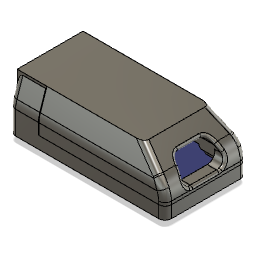
bms_can_case (Autodesk Fusion 360 design; units mm, degrees)
Autodesk Fusion 360 part; units mm, degrees
sketch "Sketch1" plane through (0, 0, 0) normal (0, 1, 0) x (1, 0, 0) in component "arduino nano"
  line L0 (0, 0) -> (44, 0)
  line L1 (44, 0) -> (44, -18)
  line L2 (44, -18) -> (0, -18)
  line L3 (0, -18) -> (0, 0)
  line L4 (0, -9) -> (-5, -9) construction
  line L5 (0, -5) -> (-5, -5)
  line L6 (0, -13) -> (-5, -13)
  line L7 (-2, -4) -> (-2, -14)
  line L8 (0, -5) -> (10, -5)
  line L9 (10, -5) -> (10, -13)
  line L10 (10, -13) -> (0, -13)
  dimension "d1571" = 44
  dimension "d1572" = 18
  dimension "d1573" = 4
  dimension "d1574" = -4
  constraint horizontal L0
  constraint vertical L1
  constraint horizontal L2
  constraint vertical L3
  constraint coincident L0.start L3.end
  constraint midpoint L3 L4.start
  constraint perpendicular L3 L4
  constraint perpendicular L6 L7
  constraint perpendicular L3 L8
  constraint perpendicular L5 L9
  measures "d1571" distance of L0.start L0.end
  measures "d1572" distance of L0.start L2.end
extrude "Extrude1" add sketch "Sketch1" along normal blind 5.7 contours L3 L8 L9 L10 | L3 L5 L6 L7 makes body 1 in component "arduino nano"
extrude "Extrude2" add sketch "Sketch1" along normal blind 1.5 contours L0 L1 L2 L3 L8 L9 L10 bodies 1 in component "arduino nano"
ref_plane "WorkPlane1" through (4, 6.2, 9) normal (0, 1, 0) x (0, 0, 1) in component "case bottom (1)"
sketch "Sketch1 (2)" plane through (4, 6.2, 9) normal (0, 1, 0) x (1, 0, 0) in component "case bottom (1)"
  line L0 (-4, 4) -> (6, 4)
  line L1 (6, 4) -> (6, -4)
  line L2 (6, -4) -> (-4, -4)
  line L3 (-4, -4) -> (-4, -9)
  line L4 (-4, -9) -> (40, -9)
  line L5 (40, -9) -> (40, 9)
  line L6 (40, 9) -> (-4, 9)
  line L7 (-4, 9) -> (-4, 4)
  line L8 (-4, 4) -> (-4, -4)
  line L9 (-8, -4) -> (-8, -13)
  line L10 (-8, -13) -> (44, -13)
  line L11 (44, -13) -> (44, 13)
  line L12 (44, 13) -> (-8, 13)
  line L13 (-8, 13) -> (-8, 4)
  line L14 (-8, 4) -> (-8, -4)
  line L15 (-4.25, -4) -> (-4.25, -9.25)
  line L16 (-4.25, -9.25) -> (40.25, -9.25)
  line L17 (40.25, -9.25) -> (40.25, 9.25)
  line L18 (40.25, 9.25) -> (-4.25, 9.25)
  line L19 (-4.25, 9.25) -> (-4.25, 4)
  line L20 (-6, 8) -> (-8, 8)
  line L21 (-6, 8) -> (-6, -8)
  line L22 (-6, -8) -> (-8, -8)
  line L23 (6, -4.5) -> (-4, -4.5) construction
  line L24 (-4, 4.5) -> (6, 4.5) construction
  line L25 (-4, 4.5) -> (-6, 4.5)
  line L26 (-4, -4.5) -> (-6, -4.5)
  dimension "d1580" = 4
  dimension "d1581" = 0.25
  dimension "d1584" = -0.5
  dimension "d1585" = -0.5
  constraint coincident L0.start L7.end
  constraint coincident L2.end L3.start
  constraint coincident L13 L20.end
  constraint perpendicular L13 L20
  constraint perpendicular L20 L21
  constraint coincident L9 L22.end
  constraint perpendicular L9 L22
  constraint coincident L21 L25.end
  constraint perpendicular L21 L25
  constraint coincident L21 L26.end
  constraint perpendicular L21 L26
extrude "Extrude1'" add sketch "Sketch1 (2)" along normal blind 0.8 separate body contours L0 L1 L2 L3 L4 L5 L6 L7 | L3 L7 L8 L21 L25 L26 | L0 L1 L2 L8 | L3 L4 L5 L6 L7 L15 L16 L17 L18 L19 L25 L26 | L9 L10 L11 L12 L13 L15 L16 L17 L18 L19 L20 L21 L22 L25 L26 makes body 2 in component "case bottom (1)"
extrude "Extrude2'" add sketch "Sketch1 (2)" against normal blind 6.5 contours L9 L10 L11 L12 L13 L15 L16 L17 L18 L19 L20 L21 L22 L25 L26 bodies 2 in component "case bottom (1)"
sketch "Sketch2" plane through (0, 6.2, 0) normal (0, -1, 0) x (1, 0, 0) in component "case bottom (1)"
  line L0 (-2, 4.5) -> (-0.25, 4.5)
  line L1 (-0.25, 4.5) -> (-0.25, -0.25)
  line L2 (-0.25, -0.25) -> (44.25, -0.25)
  line L3 (44.25, -0.25) -> (44.25, 18.25)
  line L4 (44.25, 18.25) -> (-0.25, 18.25)
  line L5 (-0.25, 18.25) -> (-0.25, 13.5)
  line L6 (-0.25, 13.5) -> (-2, 13.5)
  line L7 (-2, 13.5) -> (-2, 4.5)
  line L8 (2.25, 4.5) -> (2.25, 2.25) construction
  line L9 (2.25, 2.25) -> (41.75, 2.25) construction
  line L10 (41.75, 2.25) -> (41.75, 15.75) construction
  line L11 (41.75, 15.75) -> (2.25, 15.75) construction
  line L12 (2.25, 15.75) -> (2.25, 13.5) construction
  line L13 (2.25, 2.25) -> (2.25, -0.25)
  line L14 (2.25, 2.25) -> (-0.25, 2.25)
  line L15 (-0.25, 2.25) -> (-0.25, -0.25)
  line L16 (-0.25, -0.25) -> (2.25, -0.25)
  line L17 (2.25, 15.75) -> (-0.25, 15.75)
  line L18 (-0.25, 15.75) -> (-0.25, 18.25)
  line L19 (-0.25, 18.25) -> (2.25, 18.25)
  line L20 (2.25, 18.25) -> (2.25, 15.75)
  line L21 (41.75, 15.75) -> (44.25, 15.75)
  line L22 (44.25, 15.75) -> (44.25, 18.25)
  line L23 (44.25, 18.25) -> (41.75, 18.25)
  line L24 (41.75, 18.25) -> (41.75, 15.75)
  line L25 (41.75, 2.25) -> (44.25, 2.25)
  line L26 (44.25, 2.25) -> (44.25, -0.25)
  line L27 (44.25, -0.25) -> (41.75, -0.25)
  line L28 (41.75, -0.25) -> (41.75, 2.25)
  dimension "d1588" = -2.5
  constraint coincident L2 L13.end
  constraint perpendicular L2 L13
  constraint coincident L1 L14.end
  constraint perpendicular L1 L14
  constraint coincident L1.end L2.start
  constraint horizontal L17
  constraint vertical L18
  constraint horizontal L19
  constraint vertical L20
  constraint coincident L4.end L5.start
  constraint horizontal L21
  constraint vertical L22
  constraint horizontal L23
  constraint vertical L24
  constraint coincident L3.end L4.start
  constraint horizontal L25
  constraint vertical L26
  constraint horizontal L27
  constraint vertical L28
  constraint coincident L2.end L3.start
extrude "Extrude3" add sketch "Sketch2" along normal blind 4.5 contours L1 L2 L13 L14 L15 L16 | L4 L5 L17 L18 L19 L20 | L2 L3 L25 L26 L27 L28 | L3 L4 L21 L22 L23 L24 bodies 2 in component "case bottom (1)"
sketch "Sketch3" plane through (0, -0.3, 0) normal (0, -1, 0) x (1, 0, 0) in component "case bottom (1)"
  line L0 (-2, 17) -> (-2, 13.5)
  line L1 (-2, 13.5) -> (-0.25, 13.5)
  line L2 (-0.25, 13.5) -> (-0.25, 18.25)
  line L3 (-0.25, 18.25) -> (44.25, 18.25)
  line L4 (44.25, 18.25) -> (44.25, -0.25)
  line L5 (44.25, -0.25) -> (-0.25, -0.25)
  line L6 (-0.25, -0.25) -> (-0.25, 4.5)
  line L7 (-0.25, 4.5) -> (-2, 4.5)
  line L8 (-2, 4.5) -> (-2, 1)
  line L9 (-2, 1) -> (-4, 1)
  line L10 (-4, 1) -> (-4, -4)
  line L11 (-4, -4) -> (48, -4)
  line L12 (48, -4) -> (48, 22)
  line L13 (48, 22) -> (-4, 22)
  line L14 (-4, 22) -> (-4, 17)
  line L15 (-4, 17) -> (-2, 17)
  line L16 (9.75, 13.5) -> (9.75, 18.25) construction
  line L17 (9.75, 18.25) -> (9.75, 22)
  line L18 (9.75, 18.25) -> (9.75, -4)
  dimension "d1591" = 10
  constraint coincident L13 L17.end
  constraint perpendicular L13 L17
  constraint coincident L11 L18.end
  constraint perpendicular L11 L18
extrude "Extrude4" add sketch "Sketch3" along normal blind 4 contours L3 L4 L5 L11 L12 L13 L17 L18 bodies 2 in component "case bottom (1)"
ref_plane "WorkPlane1" through (22, -7, 9) normal (0, 1, 0) x (1, 0, 0) in component "mcp2515"
sketch "Sketch1 (3)" plane through (22, -7, 9) normal (0, 1, 0) x (1, 0, 0) in component "mcp2515"
  line L0 (-22, -9) -> (-22, 9) construction
  line L1 (-7.5, -9) -> (-7.5, 9) construction
  line L2 (-9, 0) -> (-6, 0) construction
  line L3 (-9, -13.85) -> (-6, -13.85) construction
  line L4 (-9, 13.85) -> (-6, 13.85) construction
  line L5 (-7.5, -9) -> (-7.5, -13.85) construction
  line L6 (-7.5, 9) -> (-7.5, 13.85) construction
  line L7 (-7.5, -13.85) -> (-7.5, 13.85)
  line L8 (32.5, -13.85) -> (32.5, 13.85)
  line L9 (-7.5, -13.85) -> (32.5, -13.85)
  line L10 (-7.5, 13.85) -> (32.5, 13.85)
  line L11 (-0.5, -13.85) -> (-0.5, 13.85) construction
  line L12 (5.35, -13.85) -> (5.35, 13.85) construction
  line L13 (-0.5, 0) -> (5.35, 0) construction
  line L14 (-0.5, -3.75) -> (5.35, -3.75)
  line L15 (-0.5, 3.75) -> (5.35, 3.75)
  line L16 (5.35, -3.75) -> (5.35, 3.75)
  line L17 (-0.5, -3.75) -> (-0.5, 3.75)
  line L18 (-5.5, -11.85) -> (32.5, -11.85) construction
  line L19 (-5.5, -11.85) -> (-5.5, 11.85) construction
  line L20 (-5.5, 11.85) -> (32.5, 11.85) construction
  line L21 (30.5, -13.85) -> (30.5, 13.85) construction
  circle A0 centre (30.5, -11.85) radius 1.65
  circle A1 centre (30.5, 11.85) radius 1.65
  circle A2 centre (-5.5, -11.85) radius 1.65
  circle A3 centre (-5.5, 11.85) radius 1.65
  dimension "d1595" = 14.5
  dimension "d1596" = 13.85
  dimension "d1597" = -13.85
  dimension "d1598" = 40
  dimension "d1599" = 7
  dimension "d1600" = 12.85
  dimension "d1601" = 3.75
  dimension "d1602" = -3.75
  dimension "d1603" = 2
  dimension "d1604" = 38
  dimension "d1605" = 3.3
  dimension "d1606" = 3.3
  dimension "d1607" = 3.3
  dimension "d1608" = 3.3
  constraint perpendicular L1 L2
  constraint midpoint L3 L5.end
  constraint midpoint L4 L6.end
  constraint perpendicular L3 L7
  constraint parallel L4 L10
  constraint midpoint L11 L13.start
  constraint midpoint L12 L13.end
  constraint perpendicular L12 L13
  constraint perpendicular L15 L16
  constraint perpendicular L15 L17
  constraint coincident L18 A0.centre
  constraint coincident L21 A0.centre
  constraint coincident L21 A1.centre
  constraint coincident L20 A1.centre
  constraint coincident L18.start L19.start
  constraint coincident L19.end L20.start
  measures "d1605" diameter of A0
  measures "d1606" diameter of A1
  measures "d1607" diameter of A2
  measures "d1608" diameter of A3
extrude "Extrude1''" add sketch "Sketch1 (3)" against normal blind 1.2 separate body contours L7 L8 L9 L10 | L14 L15 L16 L17 makes body 3 in component "mcp2515"
extrude "Extrude2''" add sketch "Sketch1 (3)" against normal blind 8.5 contours L14 L15 L16 L17 bodies 3 in component "mcp2515"
sketch "Sketch4" plane through (0, -4.3, 0) normal (0, -1, 0) x (1, 0, 0) in component "case bottom (1)"
  line L0 (9.75, 18.25) -> (44.25, 18.25)
  line L1 (44.25, 18.25) -> (44.25, -0.25)
  line L2 (44.25, -0.25) -> (9.75, -0.25)
  line L3 (9.75, -0.25) -> (9.75, -4)
  line L4 (9.75, -4) -> (48, -4)
  line L5 (48, -4) -> (48, 22)
  line L6 (48, 22) -> (9.75, 22)
  line L7 (9.75, 22) -> (9.75, 18.25)
  line L8 (14.5, -4.85) -> (54.5, -4.85) construction
  line L9 (14.5, 22.85) -> (14.5, -4.85) construction
  line L10 (54.5, 22.85) -> (54.5, -4.85) construction
  line L11 (14.5, 22.85) -> (54.5, 22.85) construction
  line L12 (54.75, 23.1) -> (54.75, -5.1)
  line L13 (14.25, -5.1) -> (54.75, -5.1)
  line L14 (14.25, 23.1) -> (14.25, -5.1)
  line L15 (14.25, 23.1) -> (54.75, 23.1)
  line L16 (14.5, -7.1) -> (59.5, -7.1)
  line L17 (14.5, 25.1) -> (59.5, 25.1)
  line L18 (54.5, -7.1) -> (54.5, 25.1) construction
  line L19 (59.5, -7.1) -> (59.5, 25.1)
  line L20 (9.75, 22) -> (9.75, 25.1)
  line L21 (9.75, 25.1) -> (14.5, 25.1)
  line L22 (14.25, 18.25) -> (9.75, 18.25)
  line L23 (9.75, 18.25) -> (9.75, 22)
  line L24 (14.5, -7.1) -> (9.75, -7.1)
  line L25 (9.75, -7.1) -> (9.75, -0.25)
  dimension "d1613" = 0.25
  dimension "d1616" = 5
  constraint perpendicular L17 L18
  constraint parallel L11 L17
  constraint coincident L18.end L17
  constraint parallel L8 L16
  constraint coincident L18.start L16
  constraint coincident L6.end L7.start
  constraint perpendicular L6 L20
  constraint perpendicular L7 L21
  constraint coincident L14 L22.start
  constraint coincident L0 L22.start
  constraint coincident L0.start L7.end
  constraint perpendicular L20 L24
  constraint coincident L2.end L3.start
  constraint perpendicular L2 L25
extrude "Extrude5" add sketch "Sketch4" along normal mid plane 4 contours L0 L6 L7 L14 L22 L23 | L4 L6 L12 L13 L14 L15 L16 L17 L19 L20 L21 L24 L25 | L4 L5 L6 L12 L13 L14 L15 | L2 L3 L4 L14 L25 bodies 2 in component "case bottom (1)"
extrude "Extrude6" add sketch "Sketch4" along normal blind 4 contours L0 L6 L7 L14 L22 L23 | L4 L6 L12 L13 L14 L15 L16 L17 L19 L20 L21 L24 L25 | L2 L3 L4 L14 L25 bodies 2 in component "case bottom (1)"
sketch "Sketch6" plane through (0, -7, 0) normal (0, 1, 0) x (-1, 0, 0) in component "case bottom (1)"
  circle A0 centre (-52.5, -2.85) radius 1.65
  circle A1 centre (-52.5, 20.85) radius 1.65
  circle A2 centre (-16.5, -2.85) radius 1.65
  circle A3 centre (-16.5, 20.85) radius 1.65
  line L0 (-14.5, 22.85) -> (-54.5, 22.85)
  line L1 (-54.5, 22.85) -> (-54.5, -4.85)
  line L2 (-54.5, -4.85) -> (-14.5, -4.85)
  line L3 (-14.5, -4.85) -> (-14.5, 22.85)
  circle A4 centre (-16.5, 20.85) radius 1.65 construction
  circle A5 centre (-52.5, 20.85) radius 1.65 construction
  circle A6 centre (-52.5, -2.85) radius 1.65 construction
  circle A7 centre (-16.5, -2.85) radius 1.65 construction
  line L4 (-14.25, 18.25) -> (-14.25, 23.1)
  line L5 (-14.25, 23.1) -> (-54.75, 23.1)
  line L6 (-54.75, 23.1) -> (-54.75, -5.1)
  line L7 (-54.75, -5.1) -> (-14.25, -5.1)
  line L8 (-14.25, -5.1) -> (-14.25, -0.25)
  line L9 (-14.25, 18.25) -> (-19, 18.25)
  line L10 (-19, 18.25) -> (-19, 23.1)
  line L11 (-14.25, -0.25) -> (-19, -0.25)
  line L12 (-19, -0.25) -> (-19, -5.1)
  line L13 (-49.9, 23.1) -> (-49.9, -5.1)
  line L14 (-19, 18.25) -> (-54.75, 18.25)
  line L15 (-19, -0.25) -> (-54.75, -0.25)
  circle A8 centre (-16.5, 20.85) radius 1
  circle A9 centre (-52.5, 20.85) radius 1
  circle A10 centre (-52.5, -2.85) radius 1
  circle A11 centre (-16.5, -2.85) radius 1
  dimension "d1621" = -4.85
  dimension "d1624" = 2
  dimension "d1625" = 2
  dimension "d1626" = 2
  dimension "d1627" = 2
  constraint coincident L4.start L9.start
  constraint perpendicular L3 L9
  constraint coincident L5 L10.end
  constraint perpendicular L5 L10
  constraint coincident L8.end L11.start
  constraint perpendicular L3 L11
  constraint perpendicular L2 L12
  constraint coincident L7 L12.end
  constraint coincident L6 L14.end
  constraint perpendicular L6 L14
  constraint coincident L6 L15.end
  constraint perpendicular L6 L15
  constraint concentric A4 A8
  constraint concentric A5 A9
  constraint concentric A6 A10
  constraint concentric A7 A11
  measures "d1624" diameter of A8
  measures "d1625" diameter of A9
  measures "d1626" diameter of A10
  measures "d1627" diameter of A11
extrude "Extrude7" add sketch "Sketch6" along normal blind 3.039 contours A0 | A1 | A2 | A3 | L0 L3 L9 L10 | L0 L3 L4 L5 L9 L10 | L0 L1 L13 L14 | L0 L1 L5 L6 L13 L14 | L2 L3 L7 L8 L11 L12 | L2 L3 L11 L12 | L1 L2 L13 L15 | L1 L2 L6 L7 L13 L15 | A8 | A9 | A10 | A11 bodies 2 in component "case bottom (1)"
extrude "Extrude8" cut sketch "Sketch6" along normal blind 3 contours A8 | A9 | A10 | A11 bodies 2 in component "case bottom (1)"
sketch "Sketch7" plane through (59.5, 0, 0) normal (1, 0, 0) x (0, 0, -1) in component "case bottom (1)"
  line L0 (7.1, -8.3) -> (7.1, -2.3)
  line L1 (7.1, -2.3) -> (-25.1, -2.3)
  line L2 (-25.1, -2.3) -> (-25.1, -8.3)
  line L3 (-25.1, -8.3) -> (7.1, -8.3)
  line L4 (-25.1, -2.3) -> (7.1, -2.3)
  line L5 (-22, -2.3) -> (-22, 7)
  line L6 (4, -2.3) -> (4, 7)
  line L7 (4, 7) -> (7.1, -2.3)
  line L8 (-25.1, -2.3) -> (-22, 7)
  constraint coincident L6.end L7.start
  constraint coincident L0.end L1.start
  constraint coincident L1.end L2.start
  constraint coincident L5.end L8.end
extrude "Extrude9" add sketch "Sketch7" against normal blind 49.75 contours L1 L4 L6 L7 | L1 L4 L5 L8 bodies 2 in component "case bottom (1)"
ref_plane "WorkPlane1" through (59.5, -2.3, -4) normal (0.628809, 0.77756, 0) x (-0.77756, 0.628809, 0) in component "case bottom (1)"
split "Split1" by plane through (59.5, -2.3, -4) normal (0.628809, 0.77756, 0) bodies 2 makes body 4 at (55.6667, 3.9, -5.0333) makes body 5 at (55.6667, 3.9, 23.0333) in component "case bottom (1)"
delete_body "RemoveBody1" bodies 4 in component "case bottom (1)"
delete_body "RemoveBody2" bodies 5 in component "case bottom (1)"
extrude "Extrude10" add 1 faces at (51.8333, 0.8, -4) along direction (0, 0, 1) blind 26 on bodies 2 bodies 2 in component "case bottom (1)"
sketch "Sketch8" plane through (44.25, 0, 0) normal (-1, 0, 0) x (0, 0, 1) in component "case bottom (1)"
  line L0 (2.25, 1.7) -> (-0.25, 1.7)
  line L1 (-0.25, 1.7) -> (-0.25, -4.3)
  line L2 (-0.25, -4.3) -> (18.25, -4.3)
  line L3 (18.25, -4.3) -> (18.25, 1.7)
  line L4 (18.25, 1.7) -> (15.75, 1.7)
  line L5 (15.75, 1.7) -> (15.75, 6.2)
  line L6 (15.75, 6.2) -> (2.25, 6.2)
  line L7 (2.25, 6.2) -> (2.25, 1.7)
  line L8 (15.75, 1.7) -> (2.25, 1.7)
  line L9 (-0.25, -6.3) -> (2.25, 1.7)
  line L10 (-0.25, -6.3) -> (18.25, -6.3)
  line L11 (18.25, -6.3) -> (15.75, 1.7)
  point P0 (18.25, -6.3)
  point P1 (-0.25, -6.3)
  point P2 (15.75, 1.7)
  point P3 (2.25, 1.7)
  constraint coincident P2 L4.end
  constraint coincident P3 L0.start
  constraint coincident P1 L9.start
  constraint coincident P0 L10.end
extrude "Extrude11" cut sketch "Sketch8" against normal blind 18.998 contours L2 L8 L9 L11 | L2 L9 L10 L11 bodies 2 in component "case bottom (1)"
sketch "Sketch1 (4)" plane through (0, -8.3, 0) normal (0, -1, 0) x (1, 0, 0) in component "case top (1)"
  line L0 (14.5, -7.1) -> (59.5, -7.1)
  line L1 (59.5, -7.1) -> (59.5, 25.1)
  line L2 (59.5, 25.1) -> (9.75, 25.1)
  line L3 (9.75, 25.1) -> (9.75, 22)
  line L4 (9.75, 22) -> (9.75, 18.25)
  line L5 (9.75, 18.25) -> (14.25, 18.25)
  line L6 (14.25, 18.25) -> (14.25, 23.1)
  line L7 (14.25, 23.1) -> (54.75, 23.1)
  line L8 (54.75, 23.1) -> (54.75, -5.1)
  line L9 (54.75, -5.1) -> (14.25, -5.1)
  line L10 (14.25, -5.1) -> (14.25, -0.25)
  line L11 (14.25, -0.25) -> (9.75, -0.25)
  line L12 (9.75, -0.25) -> (9.75, -7.1)
  line L13 (9.75, -7.1) -> (14.5, -7.1)
extrude "Extrude1'''" add sketch "Sketch1 (4)" along normal blind 4 separate body makes body 6 in component "case top (1)"
sketch "Sketch2 (2)" plane through (0, -12.3, 0) normal (0, -1, 0) x (1, 0, 0) in component "case top (1)"
  line L0 (9.75, -7.1) -> (14.5, -7.1)
  line L1 (14.5, -7.1) -> (59.5, -7.1)
  line L2 (59.5, -7.1) -> (59.5, 25.1)
  line L3 (59.5, 25.1) -> (9.75, 25.1)
  line L4 (9.75, 25.1) -> (9.75, 22)
  line L5 (9.75, 22) -> (9.75, 18.25)
  line L6 (9.75, 18.25) -> (14.25, 18.25)
  line L7 (14.25, 18.25) -> (14.25, 23.1)
  line L8 (14.25, 23.1) -> (54.75, 23.1)
  line L9 (54.75, 23.1) -> (54.75, -5.1)
  line L10 (54.75, -5.1) -> (14.25, -5.1)
  line L11 (14.25, -5.1) -> (14.25, -0.25)
  line L12 (14.25, -0.25) -> (9.75, -0.25)
  line L13 (9.75, -0.25) -> (9.75, -7.1)
  line L14 (27.35, 5.25) -> (27.35, 12.75)
  line L15 (27.35, 12.75) -> (21.5, 12.75)
  line L16 (21.5, 12.75) -> (21.5, 5.25)
  line L17 (21.5, 5.25) -> (27.35, 5.25)
  line L18 (28.35, 13.75) -> (20.5, 13.75)
  line L19 (20.5, 13.75) -> (20.5, 4.25)
  line L20 (20.5, 4.25) -> (28.35, 4.25)
  line L21 (28.35, 4.25) -> (28.35, 13.75)
  line L22 (9.75, 18.25) -> (9.75, -0.25)
  dimension "d1640" = 1
  constraint coincident L5.end L6.start
  constraint coincident L12.end L13.start
extrude "Extrude2'''" add sketch "Sketch2 (2)" along normal blind 0.8 contours L0 L1 L2 L3 L4 L5 L6 L7 L8 L9 L10 L11 L12 L13 | L6 L7 L8 L9 L10 L11 L12 L22 bodies 6 in component "case top (1)"
sketch "Sketch3 (2)" plane through (0, -12.3, 0) normal (0, 1, 0) x (-1, 0, 0) in component "case top (1)"
  line L0 (-14.25, -0.25) -> (-9.75, -0.25)
  line L1 (-9.75, -0.25) -> (-9.75, 18.25)
  line L2 (-9.75, 18.25) -> (-14.25, 18.25)
  line L3 (-14.25, 18.25) -> (-14.25, 23.1)
  line L4 (-14.25, 23.1) -> (-54.75, 23.1)
  line L5 (-54.75, 23.1) -> (-54.75, -5.1)
  line L6 (-54.75, -5.1) -> (-14.25, -5.1)
  line L7 (-14.25, -5.1) -> (-14.25, -0.25)
  line L8 (-28.35, 4.25) -> (-28.35, 13.75)
  line L9 (-28.35, 13.75) -> (-20.5, 13.75)
  line L10 (-20.5, 13.75) -> (-20.5, 4.25)
  line L11 (-20.5, 4.25) -> (-28.35, 4.25)
  line L12 (-14.25, -0.25) -> (-14.25, 18.25)
  constraint coincident L0.start L7.end
  constraint coincident L2.end L3.start
extrude "Extrude3'" add sketch "Sketch3 (2)" along normal blind 7 contours L0 L1 L2 L12 bodies 6 in component "case top (1)"
extrude "Extrude4'" cut 1 faces at (12.75, -6.3, 18.25) along direction (0, 0, -1) blind 0.25 on bodies 6 bodies 6 in component "case top (1)"
extrude "Extrude5'" cut 1 faces at (11.25, -6.3, -0.25) along direction (0, 0, 1) blind 0.25 on bodies 6 bodies 6 in component "case top (1)"
chamfer "Chamfer1" distance 2 distance2 3 1 edges at (14.25, -5.3, 9) measured on face at (11.25, -5.3, 12) on bodies 6 in component "case top (1)"
fillet "Fillet1" radius 3 4 edges at (34.5, -12.3, -5.1) (54.75, -12.3, 9) (34.5, -12.3, 23.1) (14.25, -12.3, 9) on bodies 6 in component "case top (1)"
sketch "Sketch4 (2)" plane through (0, -13.1, 0) normal (0, -1, 0) x (1, 0, 0) in component "case top (1)"
  line L0 (28.35, 13.75) -> (28.35, 4.25)
  line L1 (28.35, 4.25) -> (20.5, 4.25)
  line L2 (20.5, 4.25) -> (20.5, 13.75)
  line L3 (20.5, 13.75) -> (28.35, 13.75)
  line L4 (9.75, 22) -> (9.75, -7.1)
  line L5 (9.75, -7.1) -> (14.5, -7.1)
  line L6 (14.5, -7.1) -> (59.5, -7.1)
  line L7 (59.5, -7.1) -> (59.5, 25.1)
  line L8 (59.5, 25.1) -> (9.75, 25.1)
  line L9 (9.75, 25.1) -> (9.75, 22)
  line L10 (12.75, 22) -> (12.75, -4.1) construction
  line L11 (12.75, -4.1) -> (14.5, -4.1) construction
  line L12 (14.5, -4.1) -> (56.5, -4.1) construction
  line L13 (56.5, -4.1) -> (56.5, 22.1) construction
  line L14 (56.5, 22.1) -> (12.75, 22.1) construction
  line L15 (12.75, 22.1) -> (12.75, 22) construction
  circle A0 centre (12.75, 22.1) radius 2
  circle A1 centre (12.75, -4.1) radius 2
  circle A2 centre (56.5, -4.1) radius 2
  circle A3 centre (56.5, 22.1) radius 2
  circle A4 centre (12.75, 22.1) radius 1.25
  circle A5 centre (12.75, -4.1) radius 1.25
  circle A6 centre (56.5, 22.1) radius 1.25
  circle A7 centre (56.5, -4.1) radius 1.25
  dimension "d1653" = -3
  dimension "d1654" = 4
  dimension "d1655" = 4
  dimension "d1656" = 4
  dimension "d1657" = 4
  dimension "d1658" = 2.5
  dimension "d1659" = 2.5
  dimension "d1660" = 2.5
  dimension "d1661" = 2.5
  constraint coincident L14.end L15.start
  constraint coincident L10.end L11.start
  constraint coincident L12.end L13.start
  constraint coincident L13.end L14.start
  constraint concentric A0 A4
  constraint concentric A2 A7
  measures "d1654" diameter of A0
  measures "d1655" diameter of A1
  measures "d1656" diameter of A2
  measures "d1657" diameter of A3
  measures "d1658" diameter of A4
  measures "d1659" diameter of A5
  measures "d1660" diameter of A6
  measures "d1661" diameter of A7
extrude "Extrude6'" cut sketch "Sketch4 (2)" against normal blind 2 contours A0 | A1 | A2 | A3 bodies 6 in component "case top (1)"
extrude "Extrude7'" cut 4 faces at (13.1482, -13.1, 21.8612) (56.2402, -13.1, 21.65) (56.6522, -13.1, -4.3637) (12.4822, -13.1, -3.5672) along direction (0, 1, 0) blind 7.362 on bodies 6 bodies 6 in component "case top (1)"
sketch "Sketch5" plane through (9.75, 0, 0) normal (-1, 0, 0) x (0, 0, 1) in component "case top (1)"
  line L0 (0, -8.3) -> (-7.1, -8.3)
  line L1 (-7.1, -8.3) -> (-7.1, -13.1)
  line L2 (-7.1, -13.1) -> (22, -13.1)
  line L3 (22, -13.1) -> (22, -8.3)
  line L4 (22, -8.3) -> (18, -8.3)
  line L5 (18, -8.3) -> (18, -5.3)
  line L6 (18, -5.3) -> (0, -5.3)
  line L7 (0, -5.3) -> (0, -8.3)
  line L8 (25.1, -8.3) -> (22, -8.3)
  line L9 (22, -8.3) -> (22, -13.1)
  line L10 (22, -13.1) -> (25.1, -13.1)
  line L11 (25.1, -13.1) -> (25.1, -8.3)
extrude "Extrude8'" add sketch "Sketch5" along normal blind 0.25 bodies 6 in component "case top (1)"
sketch "Sketch6 (2)" plane through (9.5, 0, 0) normal (-1, 0, 0) x (0, 0, 1) in component "case top (1)"
  line L0 (25.1, -13.1) -> (25.1, -8.3)
  line L1 (25.1, -8.3) -> (18, -8.3)
  line L2 (18, -8.3) -> (18, -5.3)
  line L3 (18, -5.3) -> (0, -5.3)
  line L4 (0, -5.3) -> (0, -8.3)
  line L5 (0, -8.3) -> (-7.1, -8.3)
  line L6 (-7.1, -8.3) -> (-7.1, -13.1)
  line L7 (-7.1, -13.1) -> (25.1, -13.1)
  line L8 (-0.25, -8.3) -> (-0.25, -0.3) construction
  line L9 (-0.25, -0.3) -> (-4, -0.3) construction
  line L10 (-4, -0.3) -> (-4, 7) construction
  line L11 (-4, 7) -> (-7.1, -2.3) construction
  line L12 (-7.1, -2.3) -> (-7.1, -8.3) construction
  line L13 (-7.1, -8.3) -> (-0.25, -8.3) construction
  line L14 (25.1, -8.3) -> (25.1, -2.3) construction
  line L15 (25.1, -2.3) -> (22, -2.3) construction
  line L16 (22, -2.3) -> (22, -8.3) construction
  line L17 (22, -8.3) -> (25.1, -8.3) construction
  line L18 (22, -8.3) -> (22, -2.3) construction
  line L19 (22, -2.3) -> (25.1, -2.3) construction
  line L20 (25.1, -2.3) -> (22, 7) construction
  line L21 (22, 7) -> (22, -0.3) construction
  line L22 (22, -0.3) -> (18.25, -0.3) construction
  line L23 (18.25, -0.3) -> (18.25, -8.3) construction
  line L24 (18.25, -8.3) -> (22, -8.3) construction
  line L25 (-0.25, -0.55) -> (-4.25, -0.55) construction
  line L26 (-4.25, -0.55) -> (-4.25, 7) construction
  line L27 (22.25, 7) -> (22.25, -0.55) construction
  line L28 (22.25, -0.55) -> (18.25, -0.55) construction
  line L29 (25.1, -13.1) -> (-7.1, -13.1)
  line L30 (-7.1, -2.3) -> (-4.25, 6.25)
  line L31 (-7.1, -2.3) -> (-7.1, -13.1)
  line L32 (-4.25, 6.25) -> (-4.25, -0.55)
  line L33 (-4.25, -0.55) -> (0, -0.55)
  line L34 (0, -0.55) -> (0, -5.3)
  line L35 (25.1, -13.1) -> (25.1, -2.3)
  line L36 (25.1, -2.3) -> (22.25, 6.25)
  line L37 (22.25, 6.25) -> (22.25, -0.55)
  line L38 (22.25, -0.55) -> (18, -0.55)
  line L39 (18, -0.55) -> (18, -5.3)
  dimension "d1692" = -0.25
  dimension "d1693" = -0.25
  constraint coincident L0.start L7.end
  constraint coincident L6.end L7.start
  constraint coincident L11.end L12.start
  constraint coincident L11 L30.end
  constraint coincident L26 L30.end
  constraint perpendicular L8 L33
  constraint coincident L3.end L4.start
  constraint perpendicular L3 L34
  constraint coincident L14.end L15.start
  constraint coincident L20 L36.end
  constraint coincident L27 L36.end
  constraint perpendicular L23 L38
  constraint coincident L2.end L3.start
extrude "Extrude9'" add sketch "Sketch6 (2)" along normal blind 11.5 bodies 6 in component "case top (1)"
sketch "Sketch9" plane through (0, -8.3, 0) normal (0, -1, 0) x (1, 0, 0) in component "case bottom (1)"
  line L0 (14.5, -7.1) -> (59.5, -7.1)
  line L1 (59.5, -7.1) -> (59.5, 25.1)
  line L2 (59.5, 25.1) -> (9.75, 25.1)
  line L3 (9.75, 25.1) -> (9.75, 22)
  line L4 (9.75, 22) -> (9.75, 18.25)
  line L5 (9.75, 18.25) -> (14.25, 18.25)
  line L6 (14.25, 18.25) -> (14.25, 23.1)
  line L7 (14.25, 23.1) -> (54.75, 23.1)
  line L8 (54.75, 23.1) -> (54.75, -5.1)
  line L9 (54.75, -5.1) -> (14.25, -5.1)
  line L10 (14.25, -5.1) -> (14.25, -0.25)
  line L11 (14.25, -0.25) -> (9.75, -0.25)
  line L12 (9.75, -0.25) -> (9.75, -7.1)
  line L13 (9.75, -7.1) -> (14.5, -7.1)
  circle A0 centre (12.75, 22.1) radius 1.25 construction
  circle A1 centre (56.5, 22.1) radius 1.25 construction
  circle A2 centre (56.5, -4.1) radius 1.25 construction
  circle A3 centre (12.75, -4.1) radius 1.25 construction
  circle A4 centre (12.75, 22.1) radius 1
  circle A5 centre (12.75, -4.1) radius 1
  circle A6 centre (56.5, 22.1) radius 1
  circle A7 centre (56.5, -4.1) radius 1
  dimension "d1672" = 2
  dimension "d1673" = 2
  dimension "d1674" = 2
  dimension "d1675" = 2
  constraint concentric A0 A4
  constraint concentric A3 A5
  constraint concentric A1 A6
  constraint concentric A2 A7
  measures "d1672" diameter of A4
  measures "d1673" diameter of A5
  measures "d1674" diameter of A6
  measures "d1675" diameter of A7
extrude "Extrude12" cut sketch "Sketch9" against normal blind 4 contours A4 | A5 | A6 | A7 bodies 2 in component "case bottom (1)"
fillet "Fillet2" radius 3 2 edges at (49.4019, 1.7, 15.75) (49.4019, 1.7, 2.25) on bodies 2 in component "case bottom (1)"
fillet "Fillet3" radius 3 2 edges at (57.125, -6.3, -0.25) (57.125, -6.3, 18.25) on bodies 2 in component "case bottom (1)"
fillet "Fillet4" radius 10 5 edges at (37, -2.3, -7.1) (12.125, -2.3, -7.1) (59.5, -2.3, -3.05) (59.5, -2.3, 21.05) (34.625, -2.3, 25.1) on bodies 2 in component "case bottom (1)"
fillet "Fillet5" radius 2.5 10 edges at (59.5, -7.6869, -7.1) (59.3718, -5.4778, -7.1) (58.2593, -2.2493, -6.959) (56.5596, 0.0087, -6.3304) (51.894, 3.8509, -5.0497) (59.5, -7.6869, 25.1) (59.3718, -5.4778, 25.1) (58.2731, -2.2747, 24.9632) (56.5596, 0.0087, 24.3304) (51.894, 3.8509, 23.0497) on bodies 2 in component "case bottom (1)"
extrude "Extrude13" cut 1 faces at (-2.6667, 2.1333, 17) along direction (0, 0, 1) blind 11.404 on bodies 2 bodies 2 in component "case bottom (1)"
extrude "Extrude14" cut 1 faces at (-2.6667, 2.1333, 1) along direction (0, 0, -1) blind 11.066 on bodies 2 bodies 2 in component "case bottom (1)"
fillet "Fillet5'" radius 10 2 edges at (3.75, -2.3, -7.1) (3.75, -2.3, 25.1) on bodies 6 in component "case top (1)"
fillet "Fillet10" radius 2.5 6 edges at (-2, 2.7448, -5.4184) (-2, -2.321, -6.9709) (-2, -8.5114, -7.1) (-2, -8.5114, 25.1) (-2, -2.321, 24.9709) (-2, 2.7448, 23.4184) on bodies 6 in component "case top (1)"
fillet "Fillet11" radius 2.5 2 edges at (59.5, -10.7, -7.1) (59.5, -10.7, 25.1) on bodies 6 in component "case top (1)"
fillet "Fillet13" radius 2.5 2 edges at (3.75, -5.3, 0) (3.75, -5.3, 18) on bodies 6 in component "case top (1)"
fillet "Fillet6" radius 1 10 edges at (59.47, -6.3, 9) (59.2859, -5.0163, 16.6289) (57.7087, -1.3626, 16.7071) (56.3733, 0.1896, 16.1484) (54.8764, 1.4391, 14.7681) (54.5538, 1.7, 9) (54.8764, 1.4391, 3.2319) (56.3733, 0.1896, 1.8516) (57.7087, -1.3626, 1.2929) (59.2859, -5.0163, 1.3711) on bodies 2 in component "case bottom (1)"
fillet "Fillet14" radius 1 5 edges at (-2, -1.675, 18) (-2, -4.5678, 17.2678) (-2, -5.3, 9) (-2, -4.5678, 0.7322) (-2, -1.675, 0) on bodies 6 in component "case top (1)"
move_face "OffsetFaces1" offset -0.1 1 faces at (54.75, -7.8667, 12.0833) on bodies 2 in component "case bottom (1)"
move_face "OffsetFaces2" offset -0.1 2 faces at (14.25, -7.4333, 21.4833) (14.25, -7.8667, -1.8667) on bodies 2 in component "case bottom (1)"
component "arduino nano" placed x (1, 0, 0) y (0, 1, 0) z (0, 0, 1) at (0, 0, 0)
component "case bottom (1)" placed x (1, 0, 0) y (0, 1, 0) z (0, 0, 1) at (0, 0, 0)
component "mcp2515" placed x (1, 0, 0) y (0, 1, 0) z (0, 0, 1) at (0, 0, 0)
component "case top (1)" placed x (1, 0, 0) y (0, 1, 0) z (0, 0, 1) at (0, 0, 0)
equation "d1596 = ( 27.7 / 2 ) * 1 mm"
equation "d1597 = ( -27.7 / 2 ) * 1 mm"
equation "d1600 = 7 mm + 5.85 mm"
equation "d1601 = ( 7.5 / 2 ) * 1 mm"
equation "d1602 = ( -7.5 / 2 ) * 1 mm"
